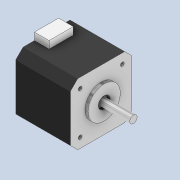
# Autodesk Inventor part: Nema 17 Stepper Motor
Saved by Autodesk Inventor 2022 (Build 260153000, 153)
## iProperties
Created: 2021-03-06
Part Number: Nema 17 Stepper Motor
Material: Generic
Document SubType Name: Modeling
Designer: Coy
Density: 1 g/cm^3
Appearance: Default(1)
Author: Coy
Autodesk Inventor part; units mm, degrees
ref_plane "YZ Plane" through (0, 0, 0) normal (1, 0, 0) x (0, 1, 0)
ref_plane "XZ Plane" through (0, 0, 0) normal (0, 1, 0) x (-1, 0, 0)
ref_plane "XY Plane" through (0, 0, 0) normal (0, 0, 1) x (1, 0, 0)
sketch "Sketch1" plane through (0, 0, 0) normal (1, 0, 0) x (0, 1, 0)
  line L0 (0, 0) -> (42, 0)
  line L1 (42, 0) -> (42, 42)
  line L2 (42, 42) -> (0, 42)
  line L3 (0, 42) -> (0, 0)
  dimension "d0" = 42
  dimension "d1" = 42
  constraints: 8 end point, 2 parallel, 1 horizontal, 1 perpendicular
  measures "d0" distance of L2.end L1.end
  measures "d1" distance of L1.end L0.end
extrude "Extrusion1" add sketch "Sketch1" against normal blind 37.25
sketch "Sketch2" plane through (0, 0, 0) normal (1, 0, 0) x (0, 0, -1)
  line L0 (-42, 42) -> (0, 42) construction
  line L1 (-21, 42) -> (-21, 0) construction
  line L2 (0, 0) -> (-42, 0) construction
  circle A0 centre (-21, 21) radius 11
  circle A1 centre (-21, 21) radius 4
  dimension "d4" = 22
  dimension "d5" = 8
  constraints: 3 midpoint, 2 centre point, 2 end point, 1 coincident
  measures "d4" diameter of A0
  measures "d5" diameter of A1
extrude "Extrusion2" add sketch "Sketch2" along normal blind 2
sketch "Sketch3" plane through (0, 21, 21) normal (1, 0, 0) x (0, 0, -1)
  circle A0 centre (0, 0) radius 4 projected
  circle A1 centre (0, 0) radius 2.5
  point P0 (21, -21)
  dimension "d8" = 5
  constraints: 1 centre point, 1 coincident
  measures "d8" diameter of A1
extrude "Extrusion3" add sketch "Sketch3" along normal blind 22 contours A1
chamfer "Chamfer1" distance 5 angle 45 4 edges at (-18.625, 42, 42) (-18.625, 42, 0) (-18.625, 0, 42) (-18.625, 0, 0)
sketch "Sketch4" plane through (0, 0, 0) normal (1, 0, 0) x (0, 0, -1)
  line L0 (-35.375, 35.3745) -> (-6.625, 35.3745) construction
  line L1 (-6.625, 35.3745) -> (-6.625, 6.6245) construction
  line L2 (-6.625, 6.6245) -> (-35.375, 6.6245) construction
  line L3 (-35.375, 6.6245) -> (-35.375, 35.3745) construction
  line L4 (-42, 37) -> (-42, 5) construction
  line L5 (-5, 42) -> (-37, 42) construction
  circle A0 centre (-6.625, 35.3745) radius 1.25
  circle A1 centre (-35.375, 35.3745) radius 1.25
  circle A2 centre (-35.375, 6.6245) radius 1.25
  circle A3 centre (-6.625, 6.6245) radius 1.25
  point P0 (0, 0)
  dimension "d14" = 28.75
  dimension "d15" = 28.75
  dimension "d16" = 6.625
  dimension "d17" = 6.6255
  dimension "d18" = 2.5
  dimension "d19" = 2.5
  dimension "d20" = 2.5
  dimension "d21" = 2.5
  constraints: 8 end point, 4 centre point, 4 coincident, 2 parallel, 1 horizontal, 1 perpendicular
  measures "d14" distance of L1.end L2.end
  measures "d15" distance of L0.end L1.end
  measures "d16" distance between parallel lines of L4 L3
  measures "d17" distance between parallel lines of L5 L0
  measures "d18" diameter of A0
  measures "d19" diameter of A1
  measures "d20" diameter of A2
  measures "d21" diameter of A3
extrude "Extrusion4" cut sketch "Sketch4" against normal blind 5
sketch "Sketch8" plane through (0, 42, 37) normal (0, 1, 0) x (1, 0, 0)
  line L0 (-37.25, 0) -> (-37.25, 32) construction
  line L1 (-37.25, 16) -> (0, 16) construction
  line L2 (0, 18.5) -> (0, 13.5) construction
  line L3 (-37.25, 7.75) -> (-27.25, 7.75)
  line L4 (-27.25, 7.75) -> (-27.25, 24.25)
  line L5 (-27.25, 24.25) -> (-37.25, 24.25)
  line L6 (-37.25, 24.25) -> (-37.25, 7.75)
  point P0 (0, 37)
  dimension "d44" = 10
  dimension "d45" = 16.5
  dimension "d46" = 8.25
  constraints: 10 end point, 2 midpoint, 2 parallel, 1 horizontal, 1 perpendicular, 1 point on line
  measures "d44" distance of L5.end L4.end
  measures "d45" distance of L4.end L3.end
  measures "d46" distance between parallel lines of L1 L5
extrude "Extrusion8" add sketch "Sketch8" along normal blind 5
equation "\"d46\" = 0.5 * d45"
body "Solid1"
